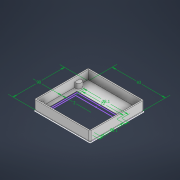
# Autodesk Inventor part: caseFront
Saved by Autodesk Inventor 2021 (Build 250183000, 183)
## iProperties
Created: 2021-08-22
Part Number: caseFront
Material: Generic
Document SubType Name: Modeling
Designer: ryanp
Density: 1 g/cm^3
Appearance: Default
Author: ryanp
Autodesk Inventor part; units mm, degrees
ref_plane "YZ Plane" through (0, 0, 0) normal (1, 0, 0) x (0, 1, 0)
ref_plane "XZ Plane" through (0, 0, 0) normal (0, 1, 0) x (-1, 0, 0)
ref_plane "XY Plane" through (0, 0, 0) normal (0, 0, 1) x (1, 0, 0)
sketch "Sketch1" plane through (0, 0, 0) normal (0, 1, 0) x (-1, 0, 0)
  line L0 (0, 0) -> (93, 0)
  line L1 (93, 0) -> (93, -90)
  line L2 (93, -90) -> (0, -90)
  line L3 (0, -90) -> (0, 0)
  line L4 (95, -92) -> (95, 2)
  line L5 (95, 2) -> (-2, 2)
  line L6 (-2, 2) -> (-2, -92)
  line L7 (-2, -92) -> (95, -92)
  line L8 (85.55, -11.63) -> (7.45, -11.63)
  line L9 (7.45, -11.63) -> (7.45, -62.73)
  line L10 (7.45, -62.73) -> (85.55, -62.73)
  line L11 (85.55, -62.73) -> (85.55, -11.63)
  line L12 (82.5, -17.18) -> (10.5, -17.18)
  line L13 (10.5, -17.18) -> (10.5, -57.18)
  line L14 (10.5, -57.18) -> (82.5, -57.18)
  line L15 (82.5, -57.18) -> (82.5, -17.18)
  arc A0 (90.8, 0) -> (93, -8.4256) centre (90.8, -4.5) ccw
  arc A1 (0, -8.4256) -> (2.2, 0) centre (2.2, -4.5) ccw
  arc A2 (93, -66.31) -> (93, -75.29) centre (90.8, -70.8) ccw
  arc A3 (0, -75.29) -> (0, -66.31) centre (2.2, -70.8) ccw
  point P0 (10.5, -37.18)
  point P1 (7.45, -37.18)
  point P2 (46.5, -62.73)
  point P3 (46.5, -57.18)
  dimension "d0" = 93
  dimension "d1" = 90
  dimension "d2" = 2
  dimension "d7" = 78.1
  dimension "d8" = 51.1
  dimension "d9" = 72
  dimension "d10" = 40
  constraints: 32 end point, 8 parallel, 8 point on circle, 8 point on line, 4 centre point, 4 coincident, 4 midpoint, 4 perpendicular, 3 horizontal, 2 tangent, 1 horizontal alignment, 1 vertical alignment, 3 other
  measures "d0" distance of L1.end L2.end
  measures "d1" distance of L0.end L1.end
  measures "d2" distance between parallel lines of L1 L4
  measures "d7" distance of L10.end L9.end
  measures "d8" distance of L9.end L8.end
  measures "d9" distance of L14.end L13.end
  measures "d10" distance of L13.end L12.end
extrude "Extrusion1" add sketch "Sketch1" along normal blind 2 contours L0 A0 L1 A2 L2 L3 A3 A1
extrude "Extrusion2" add sketch "Sketch1" along normal blind 10.5 contours L0 A1 L3 | L0 L1 A0 | A3 L3 | L1 A2
extrude "Extrusion3" add sketch "Sketch1" along normal blind 17.5 contours L7 L6 L5 L4
chamfer "Chamfer1" distance 2 angle 45 4 edges at (-46.5, 0, -11.63) (-85.55, 0, -37.18) (-7.45, 0, -37.18) (-46.5, 0, -62.73)
fillet "Fillet1" radius 2 8 edges at (-46.5, 0, -92) (2, 0, -45) (2, 8.75, -92) (-95, 8.75, -92) (-95, 0, -45) (-46.5, 0, 2) (-95, 8.75, 2) (2, 8.75, 2)
body "Solid1"
